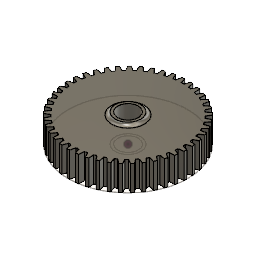
Gear v1 (Autodesk Fusion 360 design; units mm, degrees)
Autodesk Fusion 360 part; units mm, degrees
sketch "Sketch1" plane through (0, 0, 0) normal (0, 1, 0) x (1, 0, 0)
  circle A0 centre (0, 0) radius 23.5
  circle A1 centre (0, 0) radius 4
  circle A2 centre (0, 0) radius 5
  dimension "d1" = 47
  dimension "d2" = 8
  dimension "d3" = 10
  measures "d1" diameter of A0
  measures "d2" diameter of A1
  measures "d3" diameter of A2
extrude "Extrude2" add sketch "Sketch1" along normal blind 11 contours A2 makes body 1
extrude "Extrude1" add sketch "Sketch1" along normal blind 10 separate body contours A0 makes body 2
sketch "Sketch2" plane through (0, 10, 0) normal (0, 1, 0) x (-1, 0, 0)
  circle A0 centre (0, 0) radius 5
  circle A1 centre (0, 0) radius 23.5
  line L0 (0.0012, -23.5) -> (0.0012, -21.5)
  line L1 (0.0012, -23.5) -> (0.0012, -24)
  line L2 (0.0012, -21.5) -> (-0.4988, -21.5)
  line L3 (0.0012, -21.5) -> (0.5012, -21.5)
  line L4 (0.0012, -24) -> (-1.2488, -24)
  line L5 (0.0012, -24) -> (1.2512, -24)
  line L6 (1.2512, -24) -> (0.5012, -21.5)
  line L7 (-1.2488, -24) -> (-0.4988, -21.5)
  dimension "d8" = 2
  dimension "d9" = 0.5
  dimension "d10" = 0.5
  dimension "d11" = 0.5
  dimension "d12" = 1.25
  dimension "d13" = 1.25
extrude "Extrude3" cut sketch "Sketch2" against normal blind 10 contours A1 L0 L2 L7 | A1 L1 L4 L7 | A1 L1 L5 L6 | A1 L0 L3 L6 bodies 2
pattern_circular "C-Pattern1" count 45 over 360 about axis through (0, 10, 0) along (0, 1, 0) of "Extrude3"
combine "Combine1" operation add target body 2 tool bodies 1
fillet "Fillet1" radius 1.5 1 edges at (-4.6616, 10, -1.8081) on bodies 2
